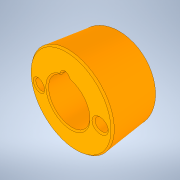
# Autodesk Inventor part: Проставка шестерни
Saved by Autodesk Inventor 2021.1 (Build 251245010, 245A)
## iProperties
Created: 2026-04-16
Part Number: Проставка шестерни
Material: Типовые
Document SubType Name: Modeling
Designer: Андрей Тарасов
Density: 1 g/cm^3
Appearance: По умолчанию
Author: Андрей Тарасов
Autodesk Inventor part; units mm, degrees
ref_plane "YZ Plane" through (0, 0, 0) normal (1, 0, 0) x (0, 1, 0)
ref_plane "XZ Plane" through (0, 0, 0) normal (0, 1, 0) x (-1, 0, 0)
ref_plane "XY Plane" through (0, 0, 0) normal (0, 0, 1) x (1, 0, 0)
sketch "Эскиз1" plane through (0, 0, 0) normal (0, 0, 1) x (1, 0, 0)
  circle A0 centre (0, 0) radius 6.1
  circle A1 centre (0, 0) radius 12
  circle A2 centre (0, 0) radius 9 construction
  line L0 (-16.8, 0) -> (16.8, 0) construction
  circle A3 centre (-9, 0) radius 1.6
  circle A4 centre (9, 0) radius 1.6
  line L1 (0, -16.8) -> (0, 16.8) construction
  circle A5 centre (0, 6.1) radius 1
  point P0 (0.9966, 6.018)
  point P1 (-0.9966, 6.018)
  dimension "d0" = 12.2
  dimension "d1" = 24
  dimension "d2" = 18
  dimension "d3" = 3.2
  dimension "d4" = 3.2
  dimension "d10" = 2
  constraints: 5 centre point, 3 coincident, 3 point on line, 2 point on circle, 3 other
  measures "d1" diameter of A1
  measures "d2" diameter of A2
  measures "d3" diameter of A3
  measures "d4" diameter of A4
  measures "d10" diameter of A5
extrude "Выдавливание1" add sketch "Эскиз1" along normal blind 13
fillet "Сопряжение1" radius 1 2 edges at (-0.9966, 6.018, 6.5) (0.9966, 6.018, 6.5)
chamfer "Фаска2" distance 0.4 angle 45 14 edges at (-1.1899, 6.105, 0) (1.1899, 6.105, 0) (0, -6.1, 0) (0, 7.1, 0) (-12, 0, 0) (7.4, 0, 0) (-10.6, 0, 0) (0, -6.1, 13) (-1.1899, 6.105, 13) (1.1899, 6.105, 13) (0, 7.1, 13) (-12, 0, 13) (-10.6, 0, 13) (7.4, 0, 13)
